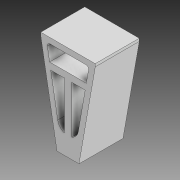
# Autodesk Inventor part: MainBracketT
Saved by Autodesk Inventor 2020 (Build 240168000, 168)
## iProperties
Created: 2021-01-14
Part Number: MainBracketT
Material: Generic
Document SubType Name: Modeling
Designer: DDeGo
Density: 1 g/cm^3
Appearance: Default
Author: DDeGo
Autodesk Inventor part; units mm, degrees
ref_plane "YZ Plane" through (0, 0, 0) normal (1, 0, 0) x (0, 1, 0)
ref_plane "XZ Plane" through (0, 0, 0) normal (0, 1, 0) x (-1, 0, 0)
ref_plane "XY Plane" through (0, 0, 0) normal (0, 0, 1) x (1, 0, 0)
sketch "Sketch1" plane through (0, 0, 0) normal (0, 0, 1) x (1, 0, 0)
  line L0 (0, 0) -> (0, 17.2417) construction
  line L1 (0, 17.2417) -> (-4.952, 17.2417)
  line L2 (-4.952, 17.2417) -> (-4.952, 16.7417)
  line L3 (-4.952, 16.7417) -> (-2, 0)
  line L4 (-2, 0) -> (0, 0)
  line L5 (0, 17.2417) -> (4.952, 17.2417)
  line L6 (4.952, 17.2417) -> (4.952, 16.7417)
  line L7 (4.952, 16.7417) -> (2, 0)
  line L8 (2, 0) -> (0, 0)
  line L9 (-3.2526, 16.2417) -> (0.4283, 16.2417)
  line L10 (0.4283, 16.2417) -> (3.2526, 16.2417)
  line L11 (3.745, 15.6549) -> (1.8611, 4.9708)
  line L12 (-1.8611, 4.9708) -> (-3.745, 15.6549)
  arc A0 (-3.2526, 16.2417) -> (-3.745, 15.6549) centre (-3.2526, 15.7417) ccw
  arc A1 (3.745, 15.6549) -> (3.2526, 16.2417) centre (3.2526, 15.7417) ccw
  arc A2 (-1.8611, 4.9708) -> (1.8611, 4.9708) centre (0, 5.299) ccw
  line L13 (-4.0013, 13.3596) -> (4.0862, 13.3596) construction
  line L14 (4.0862, 13.3596) -> (4.0862, 3.3596) construction
  line L15 (4.0862, 3.3596) -> (-4.0013, 3.3596) construction
  line L16 (-4.0013, 3.3596) -> (-4.0013, 13.3596) construction
  line L17 (-0.6545, 3.3596) -> (-0.6545, 12.1765)
  line L18 (-0.6545, 12.1765) -> (-4.0094, 12.1765)
  line L19 (-4.0094, 12.1765) -> (-4.0094, 13.3596)
  line L20 (-4.0094, 13.3596) -> (4.0295, 13.3596)
  line L21 (4.0295, 13.3596) -> (4.0295, 12.1765)
  line L22 (4.0295, 12.1765) -> (0.6746, 12.1765)
  line L23 (0.6746, 12.1765) -> (0.6746, 3.3596)
  line L24 (0.6746, 3.3596) -> (-0.6545, 3.3596)
  point P0 (-3.8484, 16.2417)
  point P1 (3.8484, 16.2417)
  point P2 (0, -5.5838)
  dimension "d0" = 2
  dimension "d1" = 10
  dimension "d2" = 0.5
  dimension "d3" = 17
  dimension "d4" = 1
  dimension "d7" = 0.5
  constraints: 26 end point, 6 point on circle, 6 point on line, 6 tangent, 3 centre point, 3 symmetric about line, 2 perpendicular, 1 equal radius, 1 parallel, 1 vertical, 5 other
  measures "d0" distance of L3.end L0.start
  measures "d1" angle of L0 L3
  measures "d2" distance of L1.end L2.end
  measures "d3" distance of L2.end L3.end
  measures "d4" distance between parallel lines of L1 L9
  measures "d7" radius of A0
extrude "Extrusion1" add sketch "Sketch1" along normal blind 8 contours L5 L6 L7 L8 L4 L3 L2 L1 | L20 L11 L22 L23 A2 L17 L18 L12 | L12 L18 L19 L20 | L20 L21 L22 L11 | A2 L23 L24 L17
body "Solid1"
